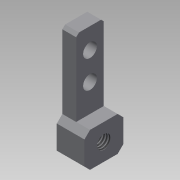
# Autodesk Inventor part: holder
Saved by Autodesk Inventor 2014 (Build 180170000, 170)
## iProperties
Created: 2013-10-11
Part Number: holder
Material: Generic
Document SubType Name: Modeling
Designer: Admin
Density: 1 g/cm^3
Appearance: Default
Author: Admin
Autodesk Inventor part; units mm, degrees
ref_plane "YZ Plane" through (0, 0, 0) normal (1, 0, 0) x (0, 1, 0)
ref_plane "XZ Plane" through (0, 0, 0) normal (0, 1, 0) x (-1, 0, 0)
ref_plane "XY Plane" through (0, 0, 0) normal (0, 0, 1) x (1, 0, 0)
sketch "Sketch1" plane through (0, 0, 0) normal (1, 0, 0) x (0, 1, 0)
  circle A0 centre (5, -7.5) radius 2.5
  circle A1 centre (5, -17.5) radius 2.5
  line L0 (0, -30) -> (10, -30)
  line L1 (10, -30) -> (10, 0)
  line L2 (10, 0) -> (0, 0)
  line L3 (0, 0) -> (0, -30)
  dimension "d23" = 30
  dimension "d25" = 30
  dimension "d38" = 10
  dimension "d39" = 5
  dimension "d40" = 5
  dimension "d41" = 10
  dimension "d42" = 5
  dimension "d43" = 5
  constraints: 8 end point, 2 centre point, 2 horizontal alignment
  measures "d23" distance of L0.start point (0, 0)
  measures "d25" distance of L1.end L0.end
  measures "d38" distance of L1.end point (0, 0)
  measures "d39" horizontal distance of point (0, 0) A0.centre
  measures "d40" horizontal distance of point (0, 0) A1.centre
  measures "d41" distance of A1.centre A0.centre
  measures "d42" diameter of A0
  measures "d43" diameter of A1
extrude "Extrusion1" add sketch "Sketch1" along normal blind 5
sketch "Sketch2" plane through (0, 0, -30) normal (0, 0, -1) x (-1, 0, 0)
  line L0 (0, 0) -> (0, 10) projected
  line L1 (0, 10) -> (-5, 10) projected
  line L2 (-5, 0) -> (-5, 10) projected
  line L3 (0, 0) -> (-5, 0) projected
extrude "Extrusion2" add sketch "Sketch2" along normal blind 10
sketch "Sketch4" plane through (0, 10, 0) normal (0, 1, 0) x (1, 0, 0)
  line L0 (5, 0) -> (5, 40) projected
  line L1 (0, 40) -> (5, 40) projected
  line L2 (0, 40) -> (5, 40)
  line L3 (5, 40) -> (5, 27.5)
  line L4 (5, 27.5) -> (0, 27.5)
  line L5 (0, 27.5) -> (0, 40)
  dimension "d5" = 12.5
  constraints: 8 end point, 2 parallel, 1 horizontal, 1 perpendicular, 1 point on line
  measures "d5" distance of L2.end L3.end
extrude "Extrusion3" add sketch "Sketch4" along normal blind 2
sketch "Sketch5" plane through (0, 0, 0) normal (0, -1, 0) x (1, 0, 0)
  line L0 (5, 0) -> (5, -40) projected
  line L1 (0, -40) -> (5, -40)
  line L2 (5, -40) -> (5, -27.5)
  line L3 (5, -27.5) -> (0, -27.5)
  line L4 (0, -27.5) -> (0, -40)
  dimension "d8" = 12.5
  constraints: 8 end point, 2 parallel, 1 horizontal, 1 perpendicular, 1 point on line
  measures "d8" distance of L2.end L1.end
extrude "Extrusion4" add sketch "Sketch5" along normal blind 2
sketch "Sketch6" plane through (5, 0, 0) normal (1, 0, 0) x (0, 0, -1)
  line L0 (27.5, 12) -> (40, 12)
  line L1 (40, 12) -> (40, -2)
  line L2 (40, -2) -> (27.5, -2)
  line L3 (27.5, -2) -> (27.5, 12)
  line L4 (40, -2) -> (40, 12) projected
  line L5 (27.5, 12) -> (40, 12) projected
  constraints: 8 end point, 2 parallel, 1 horizontal, 1 perpendicular
chamfer "Chamfer3" distance 1 angle 45 2 edges at (2.5, 10, 0) (2.5, 0, 0)
extrude "Extrusion6" add sketch "Sketch6" along normal blind 5
chamfer "Chamfer4" distance 2 angle 45 4 edges at (5, 12, -27.5) (5, 12, -40) (5, -2, -40) (5, -2, -27.5)
sketch "Sketch7" plane through (10, 0, 0) normal (1, 0, 0) x (0, 0, -1)
  line L0 (40, 0) -> (40, 10) projected
  line L1 (38, 12) -> (29.5, 12) projected
  point P0 (0, 0)
  point P1 (33.75, 5)
  dimension "d44" = 7
  dimension "d45" = 6.25
  measures "d44" distance from line of L1 point (33.75, 5)
  measures "d45" distance from line of L0 point (33.75, 5)
hole "Hole1" at (10, 5, -33.75) direction (-1, 0, 0) diameter 4.917 end through all thread size "M6x1" class "6H" standard "ISO Metric profile"
body "Solid1"
